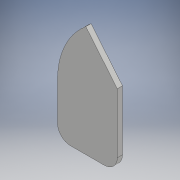
# Autodesk Inventor part: flange_small
Saved by Autodesk Inventor 2017 (Build 210142000, 142)
## iProperties
Created: 2016-09-16
Part Number: flange_small
Material: Generic
Document SubType Name: Modeling
Designer: Nic
Density: 1 g/cm^3
Appearance: Default
Author: Nic
Autodesk Inventor part; units mm, degrees
ref_plane "YZ Plane" through (0, 0, 0) normal (1, 0, 0) x (0, 1, 0)
ref_plane "XZ Plane" through (0, 0, 0) normal (0, 1, 0) x (-1, 0, 0)
ref_plane "XY Plane" through (0, 0, 0) normal (0, 0, 1) x (1, 0, 0)
sketch "Sketch1" plane through (0, 0, 0) normal (0, 1, 0) x (-1, 0, 0)
  circle A0 centre (0, 0) radius 12 construction
  line L0 (0, 0) -> (0, -50) construction
  line L1 (20, -50) -> (34, -50) construction
  line L2 (34, -50) -> (34, -16) construction
  line L3 (34, -16) -> (20, -16) construction
  line L4 (20, -16) -> (20, -50) construction
  line L5 (21, -42) -> (34, -42)
  circle A1 centre (0, 0) radius 6 construction
  line L6 (16, -14) -> (28.0909, 0.6564)
  line L7 (39, -22.4853) -> (39, -37)
  line L8 (16, -37) -> (16, -14)
  arc A2 (16, -14) -> (0, -6) centre (0, -26) ccw construction
  arc A3 (39, -22.4853) -> (28.0909, 0.6564) centre (9, -22.4853) ccw
  arc A4 (34, -42) -> (39, -37) centre (34, -37) ccw
  arc A5 (16, -37) -> (21, -42) centre (21, -37) ccw
  point P0 (16, -42)
  point P1 (39, -42)
  dimension "d26" = 12
  dimension "d0" = 50
  dimension "d1" = 24
  dimension "d16" = 16
  dimension "d17" = 34
  dimension "d18" = 23
  dimension "d19" = 26
  dimension "d21" = 5
  dimension "d23" = 20
  dimension "d25" = 16
  dimension "d27" = 30
  dimension "d28" = 19
  dimension "d30" = 5
  dimension "d31" = 5
  dimension "d32" = 20
  constraints: 18 end point, 8 point on circle, 6 point on line, 5 centre point, 5 tangent, 3 vertical, 2 horizontal, 2 parallel, 1 coincident, 1 perpendicular, 1 vertical alignment, 4 other
  measures "d0" distance of L0.start L0.end
  measures "d1" diameter of A0
  measures "d16" distance from line of point (0, 0) L3
  measures "d17" distance of L1.end L2.end
  measures "d18" distance of point (16, -42) point (39, -42)
  measures "d19" distance between parallel lines of L3 L5
  measures "d21" distance between parallel lines of L7 L2
  measures "d23" radius of A2
  measures "d25" distance from line of point (0, 0) L8
  measures "d27" radius of A3
  measures "d28" distance of L6.start L6.end
  measures "d30" radius of A4
  measures "d31" radius of A5
  measures "d32" distance between parallel lines of L0 L4
extrude "Extrusion1" add sketch "Sketch1" along normal blind 2
body "Solid1"
